Autodesk Fusion 360 part; units mm, degrees
(part 10 of 10)
equation "d2819 = TouchChamfer"
equation "d2820 = FootHeight"
equation "d2822 = ( BaseX + LeftRun + FaucetGap + ( RightRun + ModuleGap ) / 2 ) + ( ( 11 mm ) - PegSize / 2 - FitClearance )"
equation "d2823 = ( BaseY ) + ( ( 11 mm ) - PegSize / 2 - FitClearance )"
equation "d2824 = PegSize + 2 * FitClearance"
equation "d2825 = PegSize + 2 * FitClearance"
equation "d2826 = PegHeight + 0.3 mm"
equation "d2828 = FootHeight"
equation "d2830 = ( BaseX + LeftRun + FaucetGap + ( RightRun + ModuleGap ) / 2 ) + ( ( 11 mm ) - PegSize / 2 - FitClearance )"
equation "d2831 = ( BaseY ) + ( ( ( Depth ) - FrontFootInset ) - PegSize / 2 - FitClearance )"
equation "d2832 = PegSize + 2 * FitClearance"
equation "d2833 = PegSize + 2 * FitClearance"
equation "d2834 = PegHeight + 0.3 mm"
equation "d2836 = FootHeight"
equation "d2838 = ( BaseX + LeftRun + FaucetGap + ( RightRun + ModuleGap ) / 2 ) + ( ( ( ( RightRun - ModuleGap ) / 2 ) - 11 mm ) - PegSize / 2 - FitClearance )"
equation "d2839 = ( BaseY ) + ( ( 11 mm ) - PegSize / 2 - FitClearance )"
equation "d2840 = PegSize + 2 * FitClearance"
equation "d2841 = PegSize + 2 * FitClearance"
equation "d2842 = PegHeight + 0.3 mm"
equation "d2844 = FootHeight"
equation "d2846 = ( BaseX + LeftRun + FaucetGap + ( RightRun + ModuleGap ) / 2 ) + ( ( ( ( RightRun - ModuleGap ) / 2 ) - 11 mm ) - PegSize / 2 - FitClearance )"
equation "d2847 = ( BaseY ) + ( ( ( Depth ) - FrontFootInset ) - PegSize / 2 - FitClearance )"
equation "d2848 = PegSize + 2 * FitClearance"
equation "d2849 = PegSize + 2 * FitClearance"
equation "d2850 = PegHeight + 0.3 mm"
equation "d2854 = ( BaseX + LeftRun + FaucetGap + ( RightRun + ModuleGap ) / 2 ) + ( 3 mm )"
equation "d2855 = ( BaseY ) + ( 0 mm )"
equation "d2856 = RunnerWidth"
equation "d2857 = ( Depth ) - 9 mm"
equation "d2858 = FootHeight"
equation "d2862 = ( BaseX + LeftRun + FaucetGap + ( RightRun + ModuleGap ) / 2 ) + ( ( ( RightRun - ModuleGap ) / 2 ) - 3 mm - RunnerWidth )"
equation "d2863 = ( BaseY ) + ( 0 mm )"
equation "d2864 = RunnerWidth"
equation "d2865 = ( Depth ) - 9 mm"
equation "d2866 = FootHeight"
equation "d2868 = TouchChamfer"
equation "d2869 = FootHeight"
equation "d2871 = ( BaseX ) + ( ( 11 mm ) - PegSize / 2 - FitClearance )"
equation "d2872 = ( BaseY + Depth + ModuleGap ) + ( ( LeftReach ) - ( ( ( 11 mm ) - PegSize / 2 - FitClearance ) + ( PegSize + 2 * FitClearance ) ) )"
equation "d2873 = PegSize + 2 * FitClearance"
equation "d2874 = PegSize + 2 * FitClearance"
equation "d2875 = PegHeight + 0.3 mm"
equation "d2877 = FootHeight"
equation "d2879 = ( BaseX ) + ( ( ( LeftSideDepth ) - FrontFootInset ) - PegSize / 2 - FitClearance )"
equation "d2880 = ( BaseY + Depth + ModuleGap ) + ( ( LeftReach ) - ( ( ( 11 mm ) - PegSize / 2 - FitClearance ) + ( PegSize + 2 * FitClearance ) ) )"
equation "d2881 = PegSize + 2 * FitClearance"
equation "d2882 = PegSize + 2 * FitClearance"
equation "d2883 = PegHeight + 0.3 mm"
equation "d2885 = FootHeight"
equation "d2887 = ( BaseX ) + ( ( 11 mm ) - PegSize / 2 - FitClearance )"
equation "d2888 = ( BaseY + Depth + ModuleGap ) + ( ( LeftReach ) - ( ( ( ( LeftReach ) - 11 mm ) - PegSize / 2 - FitClearance ) + ( PegSize + 2 * FitClearance ) ) )"
equation "d2889 = PegSize + 2 * FitClearance"
equation "d2890 = PegSize + 2 * FitClearance"
equation "d2891 = PegHeight + 0.3 mm"
equation "d2893 = FootHeight"
equation "d2895 = ( BaseX ) + ( ( ( LeftSideDepth ) - FrontFootInset ) - PegSize / 2 - FitClearance )"
equation "d2896 = ( BaseY + Depth + ModuleGap ) + ( ( LeftReach ) - ( ( ( ( LeftReach ) - 11 mm ) - PegSize / 2 - FitClearance ) + ( PegSize + 2 * FitClearance ) ) )"
equation "d2897 = PegSize + 2 * FitClearance"
equation "d2898 = PegSize + 2 * FitClearance"
equation "d2899 = PegHeight + 0.3 mm"
equation "d2903 = ( BaseX ) + ( 0 mm )"
equation "d2904 = ( BaseY + Depth + ModuleGap ) + ( ( LeftReach ) - ( ( 3 mm ) + ( RunnerWidth ) ) )"
equation "d2905 = ( LeftSideDepth ) - 9 mm"
equation "d2906 = RunnerWidth"
equation "d2907 = FootHeight"
equation "d2911 = ( BaseX ) + ( 0 mm )"
equation "d2912 = ( BaseY + Depth + ModuleGap ) + ( ( LeftReach ) - ( ( ( LeftReach ) - 3 mm - RunnerWidth ) + ( RunnerWidth ) ) )"
equation "d2913 = ( LeftSideDepth ) - 9 mm"
equation "d2914 = RunnerWidth"
equation "d2915 = FootHeight"
equation "d2917 = TouchChamfer"
equation "d2918 = FootHeight"
equation "d2920 = ( BaseX + LeftRun + FaucetGap + RightRun - RightSideDepth ) + ( ( RightSideDepth ) - ( ( ( 11 mm ) - PegSize / 2 - FitClearance ) + ( PegSize + 2 * FitClearance ) ) )"
equation "d2921 = ( BaseY + Depth + ModuleGap ) + ( ( 11 mm ) - PegSize / 2 - FitClearance )"
equation "d2922 = PegSize + 2 * FitClearance"
equation "d2923 = PegSize + 2 * FitClearance"
equation "d2924 = PegHeight + 0.3 mm"
equation "d2926 = FootHeight"
equation "d2928 = ( BaseX + LeftRun + FaucetGap + RightRun - RightSideDepth ) + ( ( RightSideDepth ) - ( ( ( ( RightSideDepth ) - FrontFootInset ) - PegSize / 2 - FitClearance ) + ( PegSize + 2 * FitClearance ) ) )"
equation "d2929 = ( BaseY + Depth + ModuleGap ) + ( ( 11 mm ) - PegSize / 2 - FitClearance )"
equation "d2930 = PegSize + 2 * FitClearance"
equation "d2931 = PegSize + 2 * FitClearance"
equation "d2932 = PegHeight + 0.3 mm"
equation "d2934 = FootHeight"
equation "d2936 = ( BaseX + LeftRun + FaucetGap + RightRun - RightSideDepth ) + ( ( RightSideDepth ) - ( ( ( 11 mm ) - PegSize / 2 - FitClearance ) + ( PegSize + 2 * FitClearance ) ) )"
equation "d2937 = ( BaseY + Depth + ModuleGap ) + ( ( ( RightReach ) - 11 mm ) - PegSize / 2 - FitClearance )"
equation "d2938 = PegSize + 2 * FitClearance"
equation "d2939 = PegSize + 2 * FitClearance"
equation "d2940 = PegHeight + 0.3 mm"
equation "d2942 = FootHeight"
equation "d2944 = ( BaseX + LeftRun + FaucetGap + RightRun - RightSideDepth ) + ( ( RightSideDepth ) - ( ( ( ( RightSideDepth ) - FrontFootInset ) - PegSize / 2 - FitClearance ) + ( PegSize + 2 * FitClearance ) ) )"
equation "d2945 = ( BaseY + Depth + ModuleGap ) + ( ( ( RightReach ) - 11 mm ) - PegSize / 2 - FitClearance )"
equation "d2946 = PegSize + 2 * FitClearance"
equation "d2947 = PegSize + 2 * FitClearance"
equation "d2948 = PegHeight + 0.3 mm"
equation "d2952 = ( BaseX + LeftRun + FaucetGap + RightRun - RightSideDepth ) + ( ( RightSideDepth ) - ( ( 0 mm ) + ( ( RightSideDepth ) - 9 mm ) ) )"
equation "d2953 = ( BaseY + Depth + ModuleGap ) + ( 3 mm )"
equation "d2954 = ( RightSideDepth ) - 9 mm"
equation "d2955 = RunnerWidth"
equation "d2956 = FootHeight"
equation "d2960 = ( BaseX + LeftRun + FaucetGap + RightRun - RightSideDepth ) + ( ( RightSideDepth ) - ( ( 0 mm ) + ( ( RightSideDepth ) - 9 mm ) ) )"
equation "d2961 = ( BaseY + Depth + ModuleGap ) + ( ( RightReach ) - 3 mm - RunnerWidth )"
equation "d2962 = ( RightSideDepth ) - 9 mm"
equation "d2963 = RunnerWidth"
equation "d2964 = FootHeight"
equation "d2966 = TouchChamfer"
equation "d2967 = TouchChamfer"
equation "d2968 = TouchChamfer"
equation "d2969 = TouchChamfer"
equation "d2970 = TouchChamfer"
equation "d2971 = TouchChamfer"
equation "d2972 = TouchChamfer"
equation "d2973 = TouchChamfer"
named bodies: "L1_DrainPan", "L1_RemovableGrate", "L1_Foot_00", "L1_Foot_01", "L1_Foot_10", "L1_Foot_11", "L2_Integrated", "L2_RemovableGrate", "L2_Foot_00", "L2_Foot_01", "L2_Foot_10", "L2_Foot_11", "R1_Integrated", "R1_RemovableGrate", "R1_Foot_00", "R1_Foot_01", "R1_Foot_10", "R1_Foot_11", "R2_Integrated", "R2_RemovableGrate", "R2_Foot_00", "R2_Foot_01", "R2_Foot_10", "R2_Foot_11", "LS_Integrated", "LS_RemovableGrate", "LS_Foot_00", "LS_Foot_01", "LS_Foot_10", "LS_Foot_11", "RS_Integrated", "RS_RemovableGrate", "RS_Foot_00", "RS_Foot_01", "RS_Foot_10", "RS_Foot_11", "Tower_Integrated", "UP_RemovableGrate", "Tower_SideFrame_1", "Tower_SideFrame_2", "FIT_Tight", "FIT_Nominal", "FIT_Loose"
